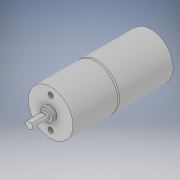
# Autodesk Inventor part: Двигун
Saved by Autodesk Inventor 2017 (Build 210142000, 142)
## iProperties
Part Number: Двигун
Material: Типовые
Document SubType Name: Modeling
Designer: Daemon
Density: 1 g/cm^3
Appearance: По умолчанию
Author: Daemon
Autodesk Inventor part; units mm, degrees
ref_plane "YZ Plane" through (0, 0, 0) normal (1, 0, 0) x (0, 1, 0)
ref_plane "XZ Plane" through (0, 0, 0) normal (0, 1, 0) x (-1, 0, 0)
ref_plane "XY Plane" through (0, 0, 0) normal (0, 0, 1) x (1, 0, 0)
sketch "Эскиз1" plane through (0, 0, 0) normal (0, 0, 1) x (1, 0, 0)
  circle A0 centre (0, 0) radius 12.5
  dimension "d0" = 25
  constraints: 1 centre point, 1 coincident
  measures "d0" diameter of A0
extrude "Выдавливание1" add sketch "Эскиз1" against normal blind 31
fillet "Сопряжение1" radius 1 1 edges at (-12.5, 0, 0)
sketch "Эскиз2" plane through (0, 0, 0) normal (0, 0, 1) x (1, 0, 0)
  circle A0 centre (0, 0) radius 12.5
  dimension "d4" = 25
  constraints: 1 centre point, 1 coincident
  measures "d4" diameter of A0
extrude "Выдавливание2" add sketch "Эскиз2" along normal blind 25
sketch "Эскиз3" plane through (0, 0, 25) normal (0, 0, 1) x (1, 0, 0)
  circle A0 centre (0, 0) radius 3.5
  dimension "d7" = 7
  constraints: 1 centre point, 1 coincident
  measures "d7" diameter of A0
extrude "Выдавливание3" add sketch "Эскиз3" along normal blind 2.5
sketch "Эскиз4" plane through (0, 0, 27.5) normal (0, 0, 1) x (1, 0, 0)
  circle A0 centre (0, 0) radius 2
  dimension "d10" = 4
  constraints: 1 centre point, 1 coincident
  measures "d10" diameter of A0
extrude "Выдавливание4" add sketch "Эскиз4" along normal blind 1.5
sketch "Эскиз5" plane through (0, 0, 29) normal (0, 0, 1) x (1, 0, 0)
  arc A0 (1.3229, -1.5) -> (-1.3229, -1.5) centre (0, 0) ccw
  line L0 (0, 0) -> (0, 2)
  line L1 (1.3229, -1.5) -> (-1.3229, -1.5)
  circle A1 centre (0, 0) radius 2 projected
  dimension "d14" = 3.5
  constraints: 4 end point, 3 point on circle, 1 centre point, 1 coincident, 1 horizontal, 1 vertical, 2 other
  measures "d14" distance from line of L1 L0.end
extrude "Выдавливание5" add sketch "Эскиз5" along normal blind 8 contours L1 A0
sketch "Эскиз6" plane through (0, 0, 25) normal (0, 0, 1) x (1, 0, 0)
  circle A0 centre (0, 0) radius 8.5
  circle A1 centre (0, -8.5) radius 1.5
  dimension "d17" = 17
  dimension "d18" = 3
  constraints: 1 centre point, 1 coincident, 1 vertical alignment, 2 other
  measures "d18" diameter of A1
extrude "Выдавливание6" cut sketch "Эскиз6" against normal blind 5 contours A1 A0 | A0 A1 picked at (0, -7.9902) picked at (0.04, -8.9886)
pattern_circular "Круговой массив1" count 2 over 360 about axis through (0, 0, 0) along (0, 0, 1) of "Выдавливание6"
